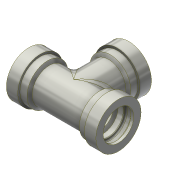
# Autodesk Inventor part: труба 3
Saved by Autodesk Inventor 2021 (Build 250183000, 183)
## iProperties
Created: 2023-02-17
Part Number: труба 3
Material: Типовые
Document SubType Name: Modeling
Designer: Tasya
Density: 1 g/cm^3
Appearance: Гладкий - слоновая кость
Author: Tasya
Autodesk Inventor part; units mm, degrees
sketch "Эскиз1" plane through (0, 0, 0) normal (0, 1, 0) x (-1, 0, 0)
  line L0 (7, 0) -> (0, 0) construction
  line L1 (0, 0) -> (0, -4) construction
  line L2 (0, -4) -> (7, -4) construction
  line L3 (7, -4) -> (7, 0) construction
  line L4 (7, 0) -> (0, 0) construction
  line L5 (0, 0) -> (0, -3.5) construction
  line L6 (0, -3.5) -> (7, -3.5) construction
  line L7 (7, -3.5) -> (7, 0) construction
  line L8 (0.64, 0) -> (0, 0) construction
  line L9 (0, 0) -> (0, -1.6667) construction
  line L10 (4, -6.5) -> (0.7, -6.5)
  line L11 (0.7, -5.9) -> (-1.366, -5.9)
  line L12 (0.7, -6.5) -> (0.7, -5.9)
  line L13 (-1.366, -5.9) -> (-1.8856, -5)
  line L14 (-1.8856, -5) -> (-8.8856, -5)
  line L15 (4, -6.5) -> (4, -4.4)
  line L16 (-0.5, -4.4) -> (-1.0196, -3.5)
  line L17 (-1.0196, -3.5) -> (-8.8856, -3.5)
  line L18 (1.6, -5) -> (2.6, -5)
  arc A0 (1.2, -4.6) -> (1.6, -5) centre (1.6, -4.6) ccw
  arc A1 (2.6, -5) -> (3, -4.6) centre (2.6, -4.6) ccw
  line L19 (4, -4.4) -> (3.2, -4.4)
  line L20 (1, -4.4) -> (-0.5, -4.4)
  arc A2 (3.2, -4.4) -> (3, -4.6) centre (3.2, -4.6) ccw
  arc A3 (1.2, -4.6) -> (1, -4.4) centre (1, -4.6) ccw
  line L21 (-8.8856, -3.5) -> (-8.8856, -0.7347) construction
  line L22 (-3.8856, -5) -> (-13.8856, -5) construction
  line L23 (-13.8856, -5) -> (-13.8856, -13.2162) construction
  line L24 (-13.8856, -13.2162) -> (-3.8856, -13.2162) construction
  line L25 (-3.8856, -13.2162) -> (-3.8856, -5) construction
  line L26 (-8.8856, -5) -> (-8.8856, -12.5) construction
  line L27 (-21.7713, -6.5) -> (-18.4713, -6.5)
  line L28 (-18.4713, -5.9) -> (-16.4053, -5.9)
  line L29 (-18.4713, -6.5) -> (-18.4713, -5.9)
  line L30 (-16.4053, -5.9) -> (-15.8856, -5)
  line L31 (-15.8856, -5) -> (-8.8856, -5)
  line L32 (-21.7713, -6.5) -> (-21.7713, -4.4)
  line L33 (-17.2713, -4.4) -> (-16.7517, -3.5)
  line L34 (-16.7517, -3.5) -> (-8.8856, -3.5)
  line L35 (-19.3713, -5) -> (-20.3713, -5)
  arc A4 (-19.3713, -5) -> (-18.9713, -4.6) centre (-19.3713, -4.6) ccw
  arc A5 (-20.7713, -4.6) -> (-20.3713, -5) centre (-20.3713, -4.6) ccw
  line L36 (-21.7713, -4.4) -> (-20.9713, -4.4)
  line L37 (-18.7713, -4.4) -> (-17.2713, -4.4)
  arc A6 (-20.7713, -4.6) -> (-20.9713, -4.4) centre (-20.9713, -4.6) ccw
  arc A7 (-18.7713, -4.4) -> (-18.9713, -4.6) centre (-18.7713, -4.6) ccw
  point P0 (1.2, -5)
  point P1 (3, -5)
  point P2 (3, -4.6)
  dimension "d14" = 1.8
  dimension "d0" = 0.5
  dimension "d1" = 4
  dimension "d2" = 7
  dimension "d6" = 5
  dimension "d9" = 1.5
  dimension "d11" = 0.4
  dimension "d12" = 0.4
  dimension "d15" = 1
  dimension "d16" = 0.4
  dimension "d17" = 1.5
  dimension "d18" = 1.5
  dimension "d19" = 1.5
  dimension "d20" = 0.2
  dimension "d21" = 0.2
  dimension "d22" = 0.5
  dimension "d23" = 4
  dimension "d24" = 0.5
  dimension "d26" = 120
  dimension "d27" = 10
  dimension "d28" = 2
  constraints: 76 end point, 20 symmetric about line, 16 point on circle, 9 parallel, 8 centre point, 7 horizontal, 6 collinear, 4 perpendicular, 4 point on line, 4 tangent, 4 vertical, 1 midpoint, 16 other
  measures "d0" distance between parallel lines of L2 L6
  measures "d1" distance between parallel lines of L2 L0
  measures "d2" distance of L0.start L0.end
  measures "d6" distance between parallel lines of L18 L0
  measures "d9" distance between parallel lines of L18 L10
  measures "d11" radius of A0
  measures "d12" radius of A1
  measures "d16" distance between parallel lines of L2 L19
  measures "d17" distance between parallel lines of L11 L20
  measures "d18" distance between parallel lines of L16 L13
  measures "d19" distance between parallel lines of L14 L17
  measures "d20" radius of A2
  measures "d21" radius of A3
  measures "d22" distance from line of A3.start L12
  measures "d23" distance between parallel lines of L1 L15
  measures "d24" distance from line of L16.start L1
  measures "d26" angle of L20 L16
  measures "d27" distance of L23.end L24.end
  measures "d28" distance from line of L25 L13.end
revolve "Вращение1" add sketch "Эскиз1" angle 360 about axis through (-7, 0, 0) along (1, 0, 0)
ref_plane "РабПлоскость2" through (8.8856, 0, 0) normal (1, 0, 0) x (0, 0, -1)
sketch "Эскиз3" plane through (8.8856, 0, 0) normal (1, 0, 0) x (0, 0, -1)
  circle A0 centre (0, 0) radius 5 projected
  line L0 (18.8856, 0) -> (11.8856, 0) construction
  line L1 (11.8856, 0) -> (11.8856, -4) construction
  line L2 (11.8856, -4) -> (18.8856, -4) construction
  line L3 (18.8856, -4) -> (18.8856, 0) construction
  line L4 (18.8856, 0) -> (11.8856, 0) construction
  line L5 (11.8856, 0) -> (11.8856, -3.5) construction
  line L6 (11.8856, -3.5) -> (18.8856, -3.5) construction
  line L7 (18.8856, -3.5) -> (18.8856, 0) construction
  line L8 (1.44, 0) -> (11.8856, 0) construction
  line L9 (11.8856, 0) -> (11.8856, -1.6667) construction
  line L10 (15.8856, -6.5) -> (12.5856, -6.5)
  line L11 (12.5856, -5.9) -> (10.5196, -5.9)
  line L12 (12.5856, -6.5) -> (12.5856, -5.9)
  line L13 (10.5196, -5.9) -> (10, -5)
  line L14 (10, -5) -> (0, -5)
  line L15 (15.8856, -6.5) -> (15.8856, -4.4)
  line L16 (11.3856, -4.4) -> (10.866, -3.5)
  line L17 (10.866, -3.5) -> (3.5707, -3.5)
  line L18 (13.4856, -5) -> (14.4856, -5)
  arc A1 (13.0856, -4.6) -> (13.4856, -5) centre (13.4856, -4.6) ccw
  line L19 (15.8856, -4.4) -> (15.0856, -4.4)
  line L20 (12.8856, -4.4) -> (11.3856, -4.4)
  arc A2 (13.0856, -4.6) -> (12.8856, -4.4) centre (12.8856, -4.6) ccw
  line L21 (11.1074, -3.5) -> (11.1074, -8.6683) construction
  line L22 (27.0859, -5) -> (17.0859, -5) construction
  line L23 (0, 0) -> (5, 0)
  circle A3 centre (0, 0) radius 5 projected
  line L24 (0, 0) -> (5, 0) construction
  arc A4 (14.4856, -5) -> (14.8856, -4.6) centre (14.4856, -4.6) ccw
  arc A5 (15.0856, -4.4) -> (14.8856, -4.6) centre (15.0856, -4.6) ccw
  point P0 (13.0856, -5)
  point P1 (14.8856, -5)
  point P2 (14.8856, -4.3091)
  point P3 (14.8856, -4.3091)
  point P4 (3, -4.6)
  point P5 (1.2, -4.6)
  point P6 (-18.9713, -4.6)
  point P7 (-20.7713, -4.6)
  point P8 (3.5707, -3.5)
  point P9 (0, -5)
  dimension "d37" = 1.8
  dimension "d30" = 0.5
  dimension "d31" = 4
  dimension "d32" = 7
  dimension "d33" = 5
  dimension "d34" = 1.5
  dimension "d35" = 0.4
  dimension "d38" = 1
  dimension "d39" = 0.4
  dimension "d40" = 1.5
  dimension "d41" = 1.5
  dimension "d42" = 1.5
  dimension "d44" = 0.2
  dimension "d45" = 0.5
  dimension "d46" = 4
  dimension "d47" = 0.5
  dimension "d48" = 120
  dimension "d51" = 0.4
  dimension "d52" = 0.2
  dimension "d53" = 10
  constraints: 50 end point, 11 point on circle, 9 horizontal, 7 collinear, 7 parallel, 4 centre point, 4 point on line, 4 tangent, 3 perpendicular, 3 vertical, 16 other
  measures "d30" distance between parallel lines of L2 L6
  measures "d31" distance between parallel lines of L2 L0
  measures "d32" distance of L0.start L0.end
  measures "d33" distance between parallel lines of L18 L0
  measures "d34" distance between parallel lines of L18 L10
  measures "d35" radius of A1
  measures "d39" distance between parallel lines of L2 L19
  measures "d40" distance between parallel lines of L11 L20
  measures "d41" distance between parallel lines of L16 L13
  measures "d42" distance between parallel lines of L14 L17
  measures "d44" radius of A2
  measures "d45" distance from line of A2.start L12
  measures "d46" distance between parallel lines of L1 L15
  measures "d47" distance from line of L16.start L1
  measures "d48" angle of L20 L16
  measures "d51" radius of A4
  measures "d52" radius of A5
  measures "d53" distance of L13.end L14.end
revolve "Вращение2" add sketch "Эскиз3" angle 360 about axis through (8.8856, 0, -1.44) along (0, 0, -1) contours A0 L17 L16 L20 A2 A1 L18 A4 A5 L19 L15 L10 L12 L11 L13 L14
sketch "Эскиз4" plane through (8.8856, 0, 0) normal (1, 0, 0) x (0, 0, -1)
  circle A0 centre (0, 0) radius 3.5
  constraints: 1 centre point, 1 coincident
hole "Отверстие1" at (8.8856, 0, 0) direction (-1, 0, 0) diameter 7 end through all both
sketch "Эскиз6" plane through (8.8856, 0, -15.8856) normal (0, 0, -1) x (-1, 0, 0)
  point P0 (8.8856, 0)
  point P1 (0, 0)
  constraints: 2 vertical alignment
hole "Отверстие2" at (8.8856, 0, -15.8856) direction (0, 0, 1) diameter 7 end up to surface
fillet "Сопряжение1" radius 2 8 edges at (12.4212, 3.5355, -3.5355) (12.4212, -3.5355, -3.5355) (5.3501, 3.5355, -3.5355) (5.3501, -3.5355, -3.5355) (11.3605, 2.4749, -2.4749) (11.3605, -2.4749, -2.4749) (6.4108, 2.4749, -2.4749) (6.4108, -2.4749, -2.4749)
ref_plane "РабПлоскость3" through (8.8856, 0, 0) normal (-1, 0, 0) x (0, 0, 1)
ref_plane "РабПлоскость4" through (0, 6.5, 0) normal (0, 1, 0) x (-1, 0, 0)
